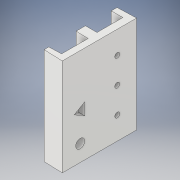
# Autodesk Inventor part: ElvDelV5
Saved by Autodesk Inventor 2019 (Build 230136000, 136)
## iProperties
Created: 2019-01-10
Part Number: ElvDelV5
Material: Acetal Resin, White
Document SubType Name: Modeling
Designer: james
Density: 1.425 g/cm^3
Appearance: Smooth - White(1)
Mass: 93.4063 g
Surface Area: 232.258 cm^2
Volume: 65.5483 cm^3
Author: james
Autodesk Inventor part; units mm, degrees
ref_plane "YZ Plane" through (0, 0, 0) normal (1, 0, 0) x (0, 1, 0)
ref_plane "XZ Plane" through (0, 0, 0) normal (0, 1, 0) x (-1, 0, 0)
ref_plane "XY Plane" through (0, 0, 0) normal (0, 0, 1) x (1, 0, 0)
sketch "Sketch1" plane through (0, 0, 0) normal (0, 1, 0) x (-1, 0, 0)
  line L0 (10.6592, 60.325) -> (-7.8828, 60.325)
  line L1 (-7.8828, 60.325) -> (-7.8828, -12.7)
  line L2 (-7.8828, -12.7) -> (10.6592, -12.7)
  line L3 (10.6592, 54.61) -> (-1.5328, 54.61)
  line L4 (-1.5328, 54.61) -> (-1.5328, 28.575)
  line L5 (-1.5328, 28.575) -> (10.6592, 28.575)
  line L6 (10.6592, 19.05) -> (-1.5328, 19.05)
  line L7 (-1.5328, 19.05) -> (-1.5328, -6.35)
  line L8 (-1.5328, -6.35) -> (10.6592, -6.35)
  line L9 (10.6592, -12.7) -> (10.6592, -6.35)
  line L10 (10.6592, 19.05) -> (10.6592, 28.575)
  line L11 (10.6592, 54.61) -> (10.6592, 60.325)
  point P0 (0, 0)
  dimension "d0" = 18.542
  dimension "d3" = 6.35
  dimension "d4" = 9.525
  dimension "d5" = 5.715
  dimension "d7" = 0
  dimension "d8" = 26.035
  dimension "d9" = 25.4
  dimension "d25" = 0
  dimension "d26" = 0
  constraints: 24 end point, 6 parallel, 3 horizontal, 3 perpendicular
  measures "d0" distance of L1.end L2.end
  measures "d3" distance between parallel lines of L2 L8
  measures "d4" distance between parallel lines of L6 L5
  measures "d5" distance between parallel lines of L0 L3
  measures "d7" distance between parallel lines of L4 L7
  measures "d8" distance of L3.end L4.end
  measures "d9" distance of L6.end L7.end
  measures "d25" distance between parallel lines of L10 L9
  measures "d26" distance between parallel lines of L10 L11
extrude "Extrusion1" add sketch "Sketch1" along normal blind 101.6
sketch "Sketch2" plane through (1.5328, 0, -6.35) normal (-1, 0, 0) x (0, 0, 1)
  line L0 (0, 0) -> (0, 101.6) projected
  line L1 (0, 0) -> (25.4, 0) projected
  point P0 (6.35, 0)
  point P1 (12.7, 25.4)
  point P2 (12.7, 50.8)
  point P3 (12.7, 76.2)
  dimension "d12" = 12.7
  dimension "d13" = 25.4
  dimension "d14" = 25.4
  dimension "d15" = 0
  dimension "d16" = 0
  dimension "d17" = 25.4
  measures "d12" distance from line of point (12.7, 25.4) L0
  measures "d13" distance from line of L1 point (12.7, 25.4)
  measures "d14" distance of point (12.7, 25.4) point (12.7, 50.8)
  measures "d15" horizontal distance of point (12.7, 25.4) point (12.7, 50.8)
  measures "d16" horizontal distance of point (12.7, 50.8) point (12.7, 76.2)
  measures "d17" distance of point (12.7, 50.8) point (12.7, 76.2)
hole "Hole1" at (1.5328, 25.4, 6.35) at (1.5328, 50.8, 6.35) at (1.5328, 76.2, 6.35) direction (1, 0, 0) diameter 4.826 depth 25.4 tip angle 118
sketch "Sketch3" plane through (0, 101.6, 0) normal (0, 1, 0) x (1, 0, 0)
  line L0 (1.5328, -28.575) -> (-10.7917, -28.1446)
  line L1 (-10.7917, -28.1446) -> (-10.7917, -28.575)
  line L2 (-10.6592, -28.575) -> (1.5328, -28.575) projected
  line L3 (-10.7917, -28.575) -> (1.5328, -28.575)
  point P0 (0, 0)
  dimension "d27" = 2
  constraints: 6 end point, 1 perpendicular, 1 vertical
  measures "d27" angle of L2 L0
extrude "Extrusion2" cut sketch "Sketch3" against normal blind 111.125
sketch "Sketch4" plane through (0, 101.6, 0) normal (0, 1, 0) x (1, 0, 0)
  line L0 (1.5328, -54.61) -> (-12.9577, -54.61)
  line L1 (-12.9577, -54.61) -> (-12.9577, -55.116)
  line L2 (-12.9577, -55.116) -> (1.5328, -54.61)
  point P0 (0, 0)
  dimension "d30" = 2
  constraints: 6 end point, 1 horizontal, 1 perpendicular
  measures "d30" angle of L2 L0
extrude "Extrusion3" cut sketch "Sketch4" against normal blind 119.0625
sketch "Sketch5" plane through (0, 101.6, 0) normal (0, 1, 0) x (1, 0, 0)
  line L0 (-10.6592, -60.325) -> (7.8828, -60.325) projected
  line L1 (7.8828, -60.325) -> (-13.0423, -59.5943)
  line L2 (-13.0423, -59.5943) -> (-13.0009, -60.325)
  line L3 (-13.0009, -60.325) -> (7.8828, -60.325)
  point P0 (0, 0)
  dimension "d33" = 2
  constraints: 6 end point, 1 collinear
  measures "d33" angle of L0 L1
extrude "Extrusion4" cut sketch "Sketch5" against normal blind 196.85
sketch "Sketch6" plane through (0, 101.6, 0) normal (0, 1, 0) x (1, 0, 0)
  line L0 (7.8828, 12.7) -> (-10.6592, 12.7) projected
  line L1 (7.8828, 12.7) -> (-16.8119, 12.7)
  line L2 (-16.8119, 12.7) -> (-16.8119, 11.8376)
  line L3 (7.8828, -60.325) -> (7.8828, 12.7) projected
  line L4 (-16.8119, 11.8376) -> (7.8828, 12.7)
  point P0 (0, 0)
  dimension "d36" = 2
  constraints: 6 end point, 1 horizontal, 1 perpendicular
  measures "d36" angle of L4 L1
extrude "Extrusion5" cut sketch "Sketch6" against normal blind 334.9625
sketch "Sketch8" plane through (1.5328, 0, -6.35) normal (-1, 0, 0) x (0, 0, 1)
  line L0 (0, 0) -> (25.4, 0) projected
  circle A0 centre (12.7, 25.4) radius 2.413 projected
  circle A1 centre (12.7, 50.8) radius 2.413 projected
  circle A2 centre (12.7, 76.2) radius 2.413 projected
  line L1 (25.4, 0) -> (25.4, 101.6) projected
  line L2 (0, 0) -> (25.4, 0)
  line L3 (25.4, 0) -> (25.4, 101.6)
  line L4 (25.4, 101.6) -> (0, 101.6)
  line L5 (0, 101.6) -> (0, 0)
  circle A3 centre (12.7, 25.4) radius 2.413
  circle A4 centre (12.7, 50.8) radius 2.413
  circle A5 centre (12.7, 76.2) radius 2.413
  point P0 (6.35, 0)
  constraints: 8 end point, 3 centre point, 3 coincident, 3 concentric, 2 parallel, 1 horizontal, 1 perpendicular
extrude "Extrusion7" add sketch "Sketch8" along normal blind 0.7937
sketch "Sketch13" plane through (1.5328, 0, 28.575) normal (-1, 0, 0) x (0, 0, 1)
  line L0 (19.995, 46.69) -> (9.7479, 40.7738)
  line L1 (9.7479, 40.7738) -> (9.7479, 52.6062)
  line L2 (9.7479, 52.6062) -> (19.995, 46.69)
  point P0 (-28.575, 0)
  point P1 (13.1636, 46.69)
  constraints: 6 end point, 7 other
extrude "Extrusion10" cut sketch "Sketch13" against normal blind 241.3
sketch "Sketch14" plane through (1.5328, 0, 28.575) normal (-1, 0, 0) x (0, 0, 1)
  circle A0 centre (14.1651, 19.3247) radius 4.4158
  point P0 (-28.575, 0)
  constraints: 1 centre point
extrude "Extrusion11" cut sketch "Sketch14" against normal blind 58.7375
sketch "Sketch15" plane through (-10.6592, 0, 19.05) normal (-1, 0, 0) x (0, 0, 1)
  line L0 (-42.6377, -21.5043) -> (50.0762, -21.5043)
  line L1 (50.0762, -21.5043) -> (50.0762, 3.175)
  line L2 (50.0762, 3.175) -> (-42.6377, 3.175)
  line L3 (-42.6377, 3.175) -> (-42.6377, -21.5043)
  line L4 (-43.9771, 109.6049) -> (47.6951, 109.6049)
  line L5 (47.6951, 109.6049) -> (47.6951, 98.425)
  line L6 (47.6951, 98.425) -> (-43.9771, 98.425)
  line L7 (-43.9771, 98.425) -> (-43.9771, 109.6049)
  line L8 (0, 101.6) -> (9.0992, 101.6) projected
  line L9 (0, 0) -> (9.0992, 0) projected
  point P0 (-19.05, 0)
  dimension "d55" = 3.175
  dimension "d56" = 3.175
  constraints: 16 end point, 4 parallel, 2 horizontal, 2 perpendicular
  measures "d55" distance between parallel lines of L6 L8
  measures "d56" distance between parallel lines of L9 L2
extrude "Extrusion12" cut sketch "Sketch15" against normal blind 58.7375
equation "\"d0\" = ElvDelWidth"
equation "\"d3\" = ElvDelFrontTabLength"
equation "\"d9\" = ElvBeamWidth"
equation "\"d10\" = ElvDelHeight"
equation "\"ElvBeamWidth\" = 25.4"
equation "\"ElvDelWidth\" = 18.542"
equation "\"ElvDelHeight\" = 101.6"
equation "\"ElvDelFrontTabLength\" = 6.35"
equation "\"ElvDelDepth\" = 6.35"
equation "\"d2\" = ElvDelDepth"
equation "\"ElvCrossBeamLength\" = 304.8"
equation "\"ElvFixedBeamLength\" = 990.6"
equation "\"ElvMiddleBeamLength\" = 990.6"
equation "\"ElvFrontBeamLength\" = 990.6"
equation "\"ElvEndEffectLength\" = 431.8"
equation "\"ElvWallWidth\" = 1.5875"
equation "\"ElvTopBeamLength\" = 457.2"
equation "\"ElvHoleFromFront\" = 25.4"
equation "\"ElvHoleFromMid\" = 38.1"
equation "\"ElvHoleFromFixed\" = 50.8"
equation "\"ElvHoleFromBottom\" = 38.1"
equation "\"ElvRivetPlateLength\" = 76.2"
equation "\"ElvDelMiddleTabLength\" = 6.35"
body "Solid1"
